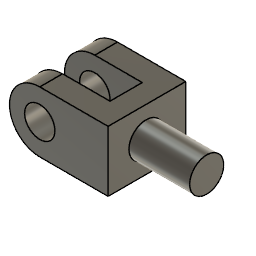
5- CREATE A 3D MODEL FROM ORTHOGRAPHIC PROJECTION (Autodesk Fusion 360 design; units mm, degrees)
part number: 2025-10-03-08-49-00-188
Autodesk Fusion 360 part; units mm, degrees
sketch "Sketch1" plane through (0, 0, 0) normal (0, 0, 1) x (1, 0, 0)
  line L0 (-90, 9) -> (-90, 20)
  line L1 (-90, 20) -> (-38, 20)
  line L2 (-38, 20) -> (-38, -20)
  line L3 (-38, -20) -> (-90, -20)
  line L4 (-90, -20) -> (-90, -9)
  line L5 (-90, -9) -> (-49, -9)
  line L6 (-49, -9) -> (-49, 9)
  line L7 (-49, 9) -> (-90, 9)
  dimension "d1" = 11
  dimension "d4" = 52
  dimension "d5" = 40
  dimension "d6" = 52
  dimension "d10" = 11
  dimension "d11" = 41
  dimension "d13" = 9
  constraint vertical L0
  constraint perpendicular L0 L1
  constraint perpendicular L1 L2
  constraint perpendicular L2 L3
  constraint perpendicular L3 L4
  constraint perpendicular L4 L5
  constraint perpendicular L5 L6
  constraint perpendicular L0 L7
  measures "d1" distance of L0.start L0.end
  measures "d4" distance of L0.end L1.end
  measures "d5" distance of L1.end L2.end
  measures "d6" distance of L2.end L3.end
  measures "d10" distance of L3.end L4.end
  measures "d11" distance of L4.end L5.end
  measures "d13" distance of origin L7
extrude "Extrude1" add sketch "Sketch1" against normal blind 32
sketch "Sketch2" plane through (-38, 0, 0) normal (1, 0, 0) x (0, 1, 0)
  line L0 (20, 0) -> (-20, 0)
  line L1 (-20, 0) -> (-20, -32)
  line L2 (-20, -32) -> (20, -32)
  line L3 (20, -32) -> (20, 0)
  circle A0 centre (0, -16) radius 9
  dimension "d16" = 18
  measures "d16" diameter of A0
extrude "Extrude2" add sketch "Sketch2" along normal blind 32 contours A0
sketch "Sketch3" plane through (0, -20, 0) normal (0, -1, 0) x (1, 0, 0)
  line L0 (-38, 0) -> (-90, 0)
  line L1 (-90, 0) -> (-90, -32)
  line L2 (-90, -32) -> (-38, -32)
  line L3 (-38, -32) -> (-38, 0)
  circle A0 centre (-74, -16) radius 8
  dimension "d19" = 16
  dimension "d20" = 36
  measures "d19" diameter of A0
  measures "d20" distance of L3 A0.centre
extrude "Extrude3" cut sketch "Sketch3" against normal blind 60 contours A0
fillet "Fillet1" radius 16 4 edges at (-90, 14.5, 0) (-90, -14.5, 0) (-90, -14.5, -32) (-90, 14.5, -32)
extrude "Extrude4" add 1 faces at (-47.3333, 20, -16) along direction (0, 1, 0) blind 1
extrude "Extrude5" add 1 faces at (-54.6667, -9, -16) along direction (0, 1, 0) blind 1
